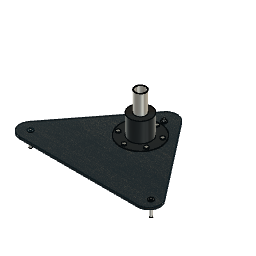
Lidar Mount (Autodesk Fusion 360 design; units mm, degrees)
Autodesk Fusion 360 part; units mm, degrees
note: some values were not read from the file. Set by a fixed rule: which face or edge a step refers to.
sketch "Sketch1" plane through (0, 0, 0) normal (0, 0, 1) x (1, 0, 0) in component "Main Mount "
  line L0 (0, 0) -> (-225, 0) construction
  line L1 (-225, 0) -> (0, 290.0012)
  line L2 (0, 290.0012) -> (225, 0)
  line L3 (-225, 0) -> (225, 0)
  dimension "d3" = 367.05
  constraint coincident L0.start origin
  constraint parallel L0 L3
  measures "d3" distance of L0.end L1.end
extrude "Extrude1" add sketch "Sketch1" along normal blind 5 makes body 1 in component "Main Mount "
fillet "Fillet1" radius 30 3 edges at (-225, 0, 2.5) (225, 0, 2.5) (0, 290.0012, 2.5) on bodies 1 in component "Main Mount "
sketch "Sketch2" plane through (0, 0, 5) normal (0, 0, 1) x (-1, 0, 0) in component "Main Mount "
  arc A0 (-23.7026, -259.4511) -> (23.7026, -259.4511) centre (0, -241.0612) ccw
  line L0 (23.7026, -259.4511) -> (187.4563, -48.3899)
  arc A1 (187.4563, -48.3899) -> (163.7537, 0) centre (163.7537, -30) ccw
  line L1 (163.7537, 0) -> (-163.7537, 0)
  arc A2 (-163.7537, 0) -> (-187.4563, -48.3899) centre (-163.7537, -30) ccw
  line L2 (-187.4563, -48.3899) -> (-23.7026, -259.4511)
  line L3 (0, -290.0012) -> (225, 0) construction
  line L4 (225, 0) -> (-225, 0) construction
  line L5 (-225, 0) -> (0, -290.0012) construction
  line L6 (0, -290.0012) -> (0, 0) construction
  circle A3 centre (0, -170) radius 55
  dimension "d8" = 110
  constraint parallel L0 L3
  constraint coincident L3 L4.start
  constraint parallel L1 L4
  constraint parallel L2 L5
  constraint coincident L6.end origin
  constraint perpendicular L1 L6
  constraint coincident L6 A3.centre
  measures "d8" diameter of A3
extrude "Extrude2" add sketch "Sketch2" along normal blind 1 separate body contours A3 makes body 2 in component "Main Mount "
sketch "Sketch3" plane through (0, 0, 6) normal (0, 0, 1) x (-1, 0, 0) in component "Main Mount "
  circle A0 centre (0, -170) radius 55
  line L0 (-5.6263, -216.2955) -> (-1.6912, -220.5202)
  line L1 (-1.6912, -220.5202) -> (3.935, -219.2248)
  line L2 (3.935, -219.2248) -> (5.6263, -213.7045)
  line L3 (5.6263, -213.7045) -> (1.6912, -209.4798)
  line L4 (1.6912, -209.4798) -> (-3.935, -210.7752)
  line L5 (-3.935, -210.7752) -> (-5.6263, -216.2955)
  line L6 (44.5974, -191.2045) -> (40.6624, -186.9798)
  line L7 (40.6624, -186.9798) -> (35.0361, -188.2752)
  line L8 (35.0361, -188.2752) -> (33.3449, -193.7955)
  line L9 (33.3449, -193.7955) -> (37.2799, -198.0202)
  line L10 (37.2799, -198.0202) -> (42.9062, -196.7248)
  line L11 (42.9062, -196.7248) -> (44.5974, -191.2045)
  line L12 (40.6624, -141.9798) -> (35.0361, -143.2752)
  line L13 (35.0361, -143.2752) -> (33.3449, -148.7955)
  line L14 (33.3449, -148.7955) -> (37.2799, -153.0202)
  line L15 (37.2799, -153.0202) -> (42.9062, -151.7248)
  line L16 (42.9062, -151.7248) -> (44.5974, -146.2045)
  line L17 (44.5974, -146.2045) -> (40.6624, -141.9798)
  line L18 (-3.935, -120.7752) -> (-5.6263, -126.2955)
  line L19 (-5.6263, -126.2955) -> (-1.6912, -130.5202)
  line L20 (-1.6912, -130.5202) -> (3.935, -129.2248)
  line L21 (3.935, -129.2248) -> (5.6263, -123.7045)
  line L22 (5.6263, -123.7045) -> (1.6912, -119.4798)
  line L23 (1.6912, -119.4798) -> (-3.935, -120.7752)
  line L24 (-44.5974, -148.7955) -> (-40.6624, -153.0202)
  line L25 (-40.6624, -153.0202) -> (-35.0361, -151.7248)
  line L26 (-35.0361, -151.7248) -> (-33.3449, -146.2045)
  line L27 (-33.3449, -146.2045) -> (-37.2799, -141.9798)
  line L28 (-37.2799, -141.9798) -> (-42.9062, -143.2752)
  line L29 (-42.9062, -143.2752) -> (-44.5974, -148.7955)
  line L30 (-40.6624, -198.0202) -> (-35.0361, -196.7248)
  line L31 (-35.0361, -196.7248) -> (-33.3449, -191.2045)
  line L32 (-33.3449, -191.2045) -> (-37.2799, -186.9798)
  line L33 (-37.2799, -186.9798) -> (-42.9062, -188.2752)
  line L34 (-42.9062, -188.2752) -> (-44.5974, -193.7955)
  line L35 (-44.5974, -193.7955) -> (-40.6624, -198.0202)
  point P0 (0, -215)
  point P1 (38.9711, -192.5)
  point P2 (38.9711, -147.5)
  point P3 (0, -125)
  point P4 (-38.9711, -147.5)
  point P5 (-38.9711, -192.5)
  dimension "d11" = 5
  dimension "d12" = 45
  dimension "d14" = 360
  measures "d11" distance of P0 L5
  measures "d12" distance of A0.centre P0
extrude "Extrude3" add sketch "Sketch3" along normal blind 2.5 separate body contours L0 L1 L2 L3 L4 L5 | L6 L7 L8 L9 L10 L11 | L12 L13 L14 L15 L16 L17 | L18 L19 L20 L21 L22 L23 | L24 L25 L26 L27 L28 L29 | L30 L31 L32 L33 L34 L35 makes body 3 at (40.2828, 146.0917, 6) makes body 4 at (-37.6595, 191.0917, 6) makes body 5 at (1.3117, 123.5917, 6) makes body 6 at (37.6595, 193.9083, 6) makes body 7 at (1.3117, 213.5917, 6) makes body 8 at (-37.6595, 146.0917, 6) in component "Main Mount "
sketch "Sketch4" plane through (0, 0, 6) normal (0, 0, 1) x (-1, 0, 0) in component "Main Mount "
  circle A0 centre (0, -170) radius 55
  circle A1 centre (0, -170) radius 30
  dimension "d17" = 60
  constraint concentric A0 A1
  measures "d17" diameter of A1
extrude "Extrude4" add sketch "Sketch4" along normal blind 54 separate body contours A1 makes body 9 in component "Main Mount "
sketch "Sketch5" plane through (0, 0, 60) normal (0, 0, 1) x (-1, 0, 0) in component "Main Mount "
  circle A0 centre (0, -170) radius 30
  circle A1 centre (0, -170) radius 15
  dimension "d20" = 30
  constraint concentric A0 A1
  measures "d20" diameter of A1
extrude "Extrude5" cut sketch "Sketch5" against normal blind 54 contours A1 bodies 9 in component "Main Mount "
sketch "Sketch6" plane through (0, 0, 60) normal (0, 0, 1) x (-1, 0, 0) in component "Main Mount "
  circle A0 centre (0, -170) radius 15
  circle A1 centre (0, -170) radius 30
  circle A2 centre (0, -170) radius 15
  constraint concentric A0 A2
extrude "Extrude6" add sketch "Sketch6" along normal blind 55 and the other way blind 54 thin wall 1.5 inside separate body contours A0 A2 makes body 10 in component "Main Mount "
sketch "Sketch7" plane through (0, 0, 5) normal (0, 0, 1) x (-1, 0, 0) in component "Main Mount "
  arc A0 (-23.7026, -259.4511) -> (23.7026, -259.4511) centre (0, -241.0612) ccw
  line L0 (23.7026, -259.4511) -> (187.4563, -48.3899)
  arc A1 (187.4563, -48.3899) -> (163.7537, 0) centre (163.7537, -30) ccw
  line L1 (163.7537, 0) -> (-163.7537, 0)
  arc A2 (-163.7537, 0) -> (-187.4563, -48.3899) centre (-163.7537, -30) ccw
  line L2 (-187.4563, -48.3899) -> (-23.7026, -259.4511)
  line L3 (-0.0023, -227.9064) -> (-6.0023, -231.3705)
  line L4 (-6.0023, -231.3705) -> (-6.0023, -238.2987)
  line L5 (-6.0023, -238.2987) -> (-0.0023, -241.7628)
  line L6 (-0.0023, -241.7628) -> (5.9977, -238.2987)
  line L7 (5.9977, -238.2987) -> (5.9977, -231.3705)
  line L8 (5.9977, -231.3705) -> (-0.0023, -227.9064)
  circle A3 centre (-0.0023, -234.8346) radius 3.5
  point P0 (-0.0023, -234.8346)
  dimension "d29" = 6
  dimension "d30" = 7
  constraint coincident P0 A3.centre
  constraint vertical L7
  measures "d29" distance of P0 L8
  measures "d30" diameter of A3
extrude "Extrude7" add sketch "Sketch7" along normal blind 2 separate body contours L3 L4 L5 L6 L7 L8 makes body 11 in component "Main Mount "
sketch "Sketch8" plane through (0, 0, 7) normal (0, 0, 1) x (-1, 0, 0) in component "Main Mount "
  circle A0 centre (-0.0023, -234.8346) radius 3.5
  line L0 (5.9977, -231.3705) -> (-0.0023, -227.9064)
  line L1 (-0.0023, -227.9064) -> (-6.0023, -231.3705)
  line L2 (-6.0023, -231.3705) -> (-6.0023, -238.2987)
  line L3 (-6.0023, -238.2987) -> (-0.0023, -241.7628)
  line L4 (-0.0023, -241.7628) -> (5.9977, -238.2987)
  line L5 (5.9977, -238.2987) -> (5.9977, -231.3705)
  circle A1 centre (-0.0023, -234.8346) radius 3.5
  dimension "d33" = 7
  constraint concentric A0 A1
  measures "d33" diameter of A1
extrude "Extrude8" add sketch "Sketch8" along normal blind 5 and the other way blind 7 separate body contours A0 A1 makes body 12 in component "Main Mount "
thread "Thread1" "ISO Metric profile 7.0 M7x0.75 6g" major diameter 6.908 minor diameter 6.0475 pitch 0.75 angle 60 resizes the face on face at (-3.4934, 235.0091, 10.3333) on face at (-3.4934, 235.0091, 2.3333) on bodies 12 in component "Main Mount "
copy_body "CopyPasteBodies1" bodies 11 12 makes body 13 makes body 14 in component "Main Mount "
move_body "Move1" bodies 13 14 to x (1, 0, 0) y (0, 1, 0) z (0, 0, 1) at (-163.5176, -205.2423, 0) in component "Main Mount "
copy_body "CopyPasteBodies2" bodies 13 14 makes body 15 makes body 16 in component "Main Mount "
move_body "Move2" bodies 15 16 to x (1, 0, 0) y (0, 1, 0) z (0, 0, 1) at (321.161, 5.5212, 0) in component "Main Mount "
sketch "Sketch9" plane through (0, 0, 5) normal (0, 0, 1) x (-1, 0, 0) in component "Main Mount "
  arc A0 (-23.7026, -259.4511) -> (23.7026, -259.4511) centre (0, -241.0612) ccw
  line L0 (23.7026, -259.4511) -> (187.4563, -48.3899)
  arc A1 (187.4563, -48.3899) -> (163.7537, 0) centre (163.7537, -30) ccw
  line L1 (163.7537, 0) -> (-163.7537, 0)
  arc A2 (-163.7537, 0) -> (-187.4563, -48.3899) centre (-163.7537, -30) ccw
  line L2 (-187.4563, -48.3899) -> (-23.7026, -259.4511)
move_body "Move3" bodies 15 16 to x (1, 0, 0) y (0, 1, 0) z (0, 0, 1) at (3.3127, -5.2034, 0) in component "Main Mount "
sketch "Sketch10" plane through (0, 0, 7) normal (0, 0, 1) x (-1, 0, 0) in component "Main Mount "
  circle A0 centre (163.5153, -29.5923) radius 3.5
  line L0 (169.5153, -26.1282) -> (163.5153, -22.6641)
  line L1 (163.5153, -22.6641) -> (157.5153, -26.1282)
  line L2 (157.5153, -26.1282) -> (157.5153, -33.0564)
  line L3 (157.5153, -33.0564) -> (163.5153, -36.5205)
  line L4 (163.5153, -36.5205) -> (169.5153, -33.0564)
  line L5 (169.5153, -33.0564) -> (169.5153, -26.1282)
move_body "Move4" bodies 16 15 to x (1, 0, 0) y (0, 1, 0) z (0, 0, 1) at (8.2887, -0.0275, 0) in component "Main Mount "
move_face "OffsetFaces1" offset -4 1 faces at (-164.0909, 28.5952, 12) on bodies 14 in component "Main Mount "
move_face "OffsetFaces2" offset -4 1 faces at (168.6714, 28.8855, 12) on bodies 16 in component "Main Mount "
sketch "Sketch11" plane through (0, 0, 0) normal (0, 0, -1) x (1, 0, 0) in component "Main Mount "
  arc A0 (-23.7026, -259.4511) -> (23.7026, -259.4511) centre (0, -241.0612) ccw
  line L0 (23.7026, -259.4511) -> (187.4563, -48.3899)
  arc A1 (187.4563, -48.3899) -> (163.7537, 0) centre (163.7537, -30) ccw
  line L1 (163.7537, 0) -> (-163.7537, 0)
  arc A2 (-163.7537, 0) -> (-187.4563, -48.3899) centre (-163.7537, -30) ccw
  line L2 (-187.4563, -48.3899) -> (-23.7026, -259.4511)
sketch "Sketch12" plane through (0, 0, 0) normal (0, 0, 1) x (1, 0, 0) in component "Main Mount "
  circle A0 centre (0, 234.8) radius 3.5
  dimension "d45" = 7
  measures "d45" diameter of A0
extrude "Extrude9" add sketch "Sketch12" against normal blind 10 separate body makes body 17 in component "Main Mount "
sketch "Sketch13" plane through (0, 0, 0) normal (0, 0, -1) x (1, 0, 0) in component "Main Mount "
  circle A0 centre (-163.5, -29.5) radius 3.5
  circle A1 centre (169.2339, -30) radius 3.5
  dimension "d48" = 7
  dimension "d49" = 7
  measures "d48" diameter of A0
  measures "d49" diameter of A1
extrude "Extrude10" add sketch "Sketch13" along normal blind 35 separate body makes body 18 at (-161.1841, 26.8758, -23.3333) makes body 19 at (165.945, 31.1971, -23.3333) in component "Main Mount "
component "Main Mount " placed x (1, 0, 0) y (0, 1, 0) z (0, 0, 1) at (0, 0, 0)
equation "d36 = 2 mm + 5 mm"
